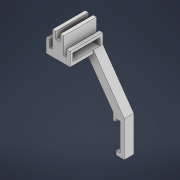
# Autodesk Inventor part: DrzakKamera
Saved by Autodesk Inventor 2022 (Build 260153000, 153)
## iProperties
Created: 2023-04-13
Part Number: DrzakKamera
Material: Všeobecné
Document SubType Name: Modeling
Designer: tada
Density: 1 g/cm^3
Appearance: Výchozí
Author: tada
Autodesk Inventor part; units mm, degrees
ref_plane "YZ Plane" through (0, 0, 0) normal (1, 0, 0) x (0, 1, 0)
ref_plane "XZ Plane" through (0, 0, 0) normal (0, 1, 0) x (-1, 0, 0)
ref_plane "XY Plane" through (0, 0, 0) normal (0, 0, 1) x (1, 0, 0)
sketch "Náčrt1" plane through (0, 0, 0) normal (0, 0, 1) x (1, 0, 0)
  line L0 (21, 22) -> (21, -30)
  line L1 (21, -30) -> (8.9, -30)
  line L2 (8.9, -30) -> (8.9, -24)
  line L3 (8.9, -24) -> (15, -24)
  line L4 (15, -24) -> (15, 16)
  line L5 (15, 16) -> (8.9, 16)
  line L6 (8.9, 16) -> (8.9, 12)
  line L7 (8.9, 12) -> (4.9, 12)
  line L8 (4.9, 12) -> (4.9, 22)
  line L9 (4.9, 22) -> (-37.1125, 82)
  line L10 (-24.5135, 87) -> (21, 22)
  line L11 (-37.1125, 82) -> (-59.5135, 82)
  line L12 (-59.5135, 82) -> (-59.5135, 87)
  line L13 (-59.5135, 87) -> (-24.5135, 87)
  point P0 (0, 0)
  dimension "d10" = 40
  dimension "d14" = 6.1
  dimension "d15" = 4
  dimension "d16" = 4
  dimension "d28" = 6
  dimension "d29" = 12.1
  dimension "d30" = 6
  dimension "d31" = 6.1
  dimension "d32" = 145
  dimension "d33" = 15
  dimension "d34" = 145
  dimension "d35" = 52
  dimension "d36" = 10
  dimension "d37" = 30
  dimension "d40" = 60
  dimension "d41" = 65
  dimension "d43" = 35
  dimension "d44" = 5
  constraints: 28 end point, 9 perpendicular, 1 horizontal, 1 parallel, 1 point on line
  measures "d10" distance between parallel lines of L5 L3
  measures "d14" distance of L4.end L5.end
  measures "d15" distance of L5.end L6.end
  measures "d16" distance of L6.end L7.end
  measures "d28" distance between parallel lines of L4 L0
  measures "d29" distance of L0.end L1.end
  measures "d30" distance of L1.end L2.end
  measures "d31" distance of L2.end L3.end
  measures "d32" angle of L9 L8
  measures "d33" distance from line of point (0, 0) L4
  measures "d34" angle of L10 L0
  measures "d35" distance of L0.start L0.end
  measures "d36" distance of L7.end L8.end
  measures "d37" distance from line of point (0, 0) L1
  measures "d40" vertical distance of L8.end L9.end
  measures "d41" vertical distance of L10.start L0.start
  measures "d43" distance of L12.end L10.start
  measures "d44" distance of L11.end L12.end
extrude "Vysunutí1" add sketch "Náčrt1" along normal blind 6 and the other way blind 4
sketch "Náčrt2" plane through (0, 0, 6) normal (0, 0, 1) x (1, 0, 0)
  line L0 (-59.5135, 82) -> (-37.1125, 82) projected
  line L1 (-24.5135, 87) -> (-59.5135, 87) projected
  line L2 (-59.5135, 82) -> (-24.5135, 82)
  line L3 (-24.5135, 82) -> (-24.5135, 87)
  line L4 (-24.5135, 87) -> (-59.5135, 87)
  line L5 (-59.5135, 87) -> (-59.5135, 82)
  point P0 (0, 0)
  constraints: 8 end point, 2 parallel, 1 horizontal, 1 perpendicular
extrude "Vysunutí2" add sketch "Náčrt2" along normal blind 30
sketch "Náčrt3" plane through (-59.5135, 87, -4) normal (0, 1, 0) x (1, 0, 0)
  circle A0 centre (17, -19) radius 3.75
  line L0 (0, 0) -> (35, 0) projected
  line L1 (35, -10) -> (35, -40) projected
  point P0 (59.5135, -4)
  dimension "d49" = 7.5
  dimension "d50" = 19
  dimension "d51" = 18
  constraints: 1 centre point
  measures "d49" diameter of A0
  measures "d50" distance from line of L0 A0.centre
  measures "d51" distance from line of L1 A0.centre
extrude "Vysunutí3" cut sketch "Náčrt3" against normal blind 30
sketch "Náčrt4" plane through (-59.5135, 82, -4) normal (0, -1, 0) x (1, 0, 0)
  line L0 (0, 40) -> (35, 40) projected
  line L1 (35, 40) -> (0, 40)
  line L2 (0, 40) -> (0, 44)
  line L3 (0, 44) -> (35, 44)
  line L4 (35, 44) -> (35, 40)
  line L5 (0, 0) -> (35, 0)
  line L6 (35, 0) -> (35, -4)
  line L7 (35, -4) -> (0, -4)
  line L8 (0, -4) -> (0, 0)
  line L9 (22.401, 0) -> (0, 0) projected
  point P0 (59.5135, 4)
  dimension "d54" = 4
  dimension "d55" = 4
  dimension "d57" = 35
  dimension "d58" = 35
  constraints: 16 end point, 4 parallel, 2 horizontal, 2 perpendicular, 1 collinear, 1 point on line
  measures "d54" distance of L3.end L0.end
  measures "d55" distance of L5.end L6.end
  measures "d57" distance of L2.end L3.end
  measures "d58" distance of L6.end L7.end
extrude "Vysunutí4" add sketch "Náčrt4" against normal blind 16
sketch "Náčrt5" plane through (-59.5135, 82, 40) normal (0, 0, 1) x (1, 0, 0)
  line L0 (0, 16) -> (35, 16) projected
  line L1 (0, 16) -> (35, 16)
  line L2 (35, 16) -> (35, 20)
  line L3 (35, 20) -> (0, 20)
  line L4 (0, 20) -> (0, 16)
  point P0 (59.5135, -82)
  dimension "d61" = 35
  dimension "d62" = 4
  constraints: 8 end point, 2 parallel, 1 horizontal, 1 perpendicular
  measures "d61" distance of L2.end L3.end
  measures "d62" distance of L1.end L2.end
extrude "Vysunutí5" add sketch "Náčrt5" against normal blind 48
sketch "Náčrt6" plane through (-59.5135, 82, 40) normal (0, 0, 1) x (1, 0, 0)
  line L0 (5, 20) -> (9.2, 20)
  line L1 (9.2, 20) -> (9.2, 10)
  line L2 (9.2, 10) -> (5, 10)
  line L3 (5, 10) -> (5, 20)
  line L4 (25.8, 20) -> (30, 20)
  line L5 (30, 20) -> (30, 10)
  line L6 (30, 10) -> (25.8, 10)
  line L7 (25.8, 10) -> (25.8, 20)
  line L8 (35, 20) -> (0, 20) projected
  line L9 (0, 0) -> (0, 20) projected
  line L10 (35, 0) -> (35, 20) projected
  point P0 (59.5135, -82)
  dimension "d65" = 5
  dimension "d66" = 4.2
  dimension "d67" = 5
  dimension "d68" = 4.2
  dimension "d69" = 10
  dimension "d70" = 10
  constraints: 16 end point, 4 parallel, 2 collinear, 2 horizontal, 2 perpendicular
  measures "d65" distance between parallel lines of L9 L3
  measures "d66" distance of L0.start L0.end
  measures "d67" distance between parallel lines of L10 L5
  measures "d68" distance of L4.start L4.end
  measures "d69" distance of L4.end L5.end
  measures "d70" distance of L2.end L0.start
extrude "Vysunutí6" cut sketch "Náčrt6" against normal blind 50
sketch "Náčrt8" plane through (-50.3135, 102, 40) normal (0, 1, 0) x (1, 0, 0)
  line L0 (0, 48) -> (0, 0) projected
  line L1 (16.6, 0) -> (0, 0) projected
  line L2 (0, 48) -> (16.6, 48)
  line L3 (16.6, 48) -> (16.6, 0)
  line L4 (16.6, 0) -> (0, 0)
  line L5 (0, 0) -> (0, 48)
  point P0 (50.3135, 40)
  constraints: 8 end point, 2 parallel, 1 horizontal, 1 perpendicular
extrude "Vysunutí7" add sketch "Náčrt8" along normal blind 5
sketch "Náčrt9" plane through (-50.3135, 107, 40) normal (0, 1, 0) x (1, 0, 0)
  line L0 (0, 48) -> (0, 0) projected
  line L1 (25.8, 0) -> (-9.2, 0) projected
  line L2 (0, 48) -> (5, 48)
  line L3 (5, 48) -> (5, 0)
  line L4 (5, 0) -> (0, 0)
  line L5 (0, 0) -> (0, 48)
  line L6 (16.6, 48) -> (11.6, 48)
  line L7 (11.6, 48) -> (11.6, 0)
  line L8 (11.6, 0) -> (16.6, 0)
  line L9 (16.6, 0) -> (16.6, 48)
  point P0 (50.3135, 40)
  point P1 (16.6, 0)
  dimension "d75" = 5
  dimension "d76" = 5
  constraints: 16 end point, 4 parallel, 2 horizontal, 2 perpendicular, 2 point on line
  measures "d75" distance of L0.start L2.end
  measures "d76" distance of L6.start L6.end
extrude "Vysunutí8" add sketch "Náčrt9" along normal blind 10
sketch "Náčrt11" plane through (0, 0, -4) normal (0, 0, -1) x (-1, 0, 0)
  line L0 (37.1125, 82) -> (-4.9, 22) projected
  line L1 (37.1125, 82) -> (-4.9, 22)
  line L2 (-4.9, 22) -> (-4.9, 12) projected
  line L3 (-4.9, 22) -> (-4.9, 12)
  line L4 (-4.9, 12) -> (-8.9, 12) projected
  line L5 (-4.9, 12) -> (-8.9, 12)
  line L6 (-8.9, 12) -> (-8.9, 16) projected
  line L7 (-8.9, 12) -> (-8.9, 16)
  line L8 (-8.9, 16) -> (-15, 16) projected
  line L9 (-8.9, 16) -> (-15, 16)
  line L10 (-15, 16) -> (-15, -24) projected
  line L11 (-15, 16) -> (-15, -24)
  line L12 (-15, -24) -> (-8.9, -24) projected
  line L13 (-15, -24) -> (-8.9, -24)
  line L14 (-8.9, -24) -> (-8.9, -30) projected
  line L15 (-8.9, -24) -> (-8.9, -30)
  line L16 (-8.9, -30) -> (-21, -30) projected
  line L17 (-8.9, -30) -> (-21, -30)
  line L18 (-21, -30) -> (-21, 22) projected
  line L19 (-21, -30) -> (-21, 22)
  line L20 (24.5135, 87) -> (59.5135, 87) projected
  line L21 (-21, 22) -> (24.5135, 87)
  line L22 (24.5135, 82) -> (24.5135, 102) projected
  line L23 (24.5135, 87) -> (24.5135, 82)
  line L24 (24.5135, 82) -> (37.1125, 82)
  line L25 (24.5135, 82) -> (59.5135, 82) projected
  point P0 (0, 0)
  constraints: 26 end point, 7 collinear, 5 perpendicular, 1 parallel
extrude "Vysunutí9" add sketch "Náčrt11" along normal blind 4
